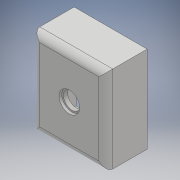
# Autodesk Inventor part: cover
Saved by Autodesk Inventor 2018 (Build 220112000, 112)
## iProperties
Created: 2019-05-15
Part Number: cover
Material: Generic
Document SubType Name: Modeling
Designer: jstklein
Density: 1 g/cm^3
Appearance: Default
Author: jstklein
Autodesk Inventor part; units mm, degrees
ref_plane "YZ Plane" through (0, 0, 0) normal (1, 0, 0) x (0, 1, 0)
ref_plane "XZ Plane" through (0, 0, 0) normal (0, 1, 0) x (-1, 0, 0)
ref_plane "XY Plane" through (0, 0, 0) normal (0, 0, 1) x (1, 0, 0)
sketch "Sketch1" plane through (0, 0, 0) normal (0, 1, 0) x (-1, 0, 0)
  line L0 (26.5, 31.5) -> (-26.5, 31.5)
  line L1 (-26.5, 31.5) -> (-26.5, -31.5)
  line L2 (-26.5, -31.5) -> (26.5, -31.5)
  line L3 (26.5, -31.5) -> (26.5, 31.5)
  line L4 (26.5, 31.5) -> (-26.5, -31.5) construction
  line L5 (-26.5, 31.5) -> (26.5, -31.5) construction
  point P0 (0, 0)
  dimension "d0" = 53
  dimension "d1" = 63
  constraints: 12 end point, 2 midpoint, 2 parallel, 1 horizontal, 1 perpendicular
  measures "d0" distance of L2.end L1.end
  measures "d1" distance of L1.end L0.end
extrude "Extrusion1" add sketch "Sketch1" along normal blind 30
sketch "Sketch2" plane through (0, 30, 0) normal (0, 1, 0) x (1, 0, 0)
  line L0 (-25, -30) -> (25, -30)
  line L1 (25, -30) -> (25, 30)
  line L2 (25, 30) -> (-25, 30)
  line L3 (-25, 30) -> (-25, -30)
  line L4 (-25, -30) -> (25, 30) construction
  line L5 (25, -30) -> (-25, 30) construction
  point P0 (0, 0)
  dimension "d4" = 50
  dimension "d5" = 60
  constraints: 12 end point, 2 midpoint, 2 parallel, 1 horizontal, 1 perpendicular
  measures "d4" distance of L2.end L1.end
  measures "d5" distance of L1.end L0.end
extrude "Extrusion2" cut sketch "Sketch2" against normal blind 25
sketch "Sketch3" plane through (0, 0, 0) normal (0, -1, 0) x (1, 0, 0)
  line L0 (26.5, -31.5) -> (-26.5, -31.5) projected
  circle A0 centre (0, 0) radius 7.5
  dimension "d10" = 15
  constraints: 1 centre point, 1 coincident
  measures "d10" diameter of A0
extrude "Extrusion3" cut sketch "Sketch3" against normal blind 2
sketch "Sketch4" plane through (0, 2, 0) normal (0, -1, 0) x (1, 0, 0)
  circle A0 centre (0, 0) radius 6.25
  dimension "d13" = 12.5
  constraints: 1 centre point, 1 coincident
  measures "d13" diameter of A0
extrude "Extrusion4" cut sketch "Sketch4" against normal up to next
fillet "Fillet1" radius 5 4 edges at (-26.5, 0, 0) (0, 0, 31.5) (26.5, 0, 0) (0, 0, -31.5)
body "Solid1"
